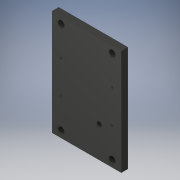
# Autodesk Inventor part: lidarCamMount
Saved by Autodesk Inventor 2017 (Build 210142000, 142)
## iProperties
Created: 2017-03-03
Part Number: lidarCamMount
Material: Polyethylene, High Density
Document SubType Name: Modeling
Designer: Naga
Density: 0.952 g/cm^3
Appearance: Smooth - Black
Author: Naga
Autodesk Inventor part; units mm, degrees
ref_plane "YZ Plane" through (0, 0, 0) normal (1, 0, 0) x (0, 1, 0)
ref_plane "XZ Plane" through (0, 0, 0) normal (0, 1, 0) x (-1, 0, 0)
ref_plane "XY Plane" through (0, 0, 0) normal (0, 0, 1) x (1, 0, 0)
sketch "Sketch1" plane through (0, 0, 0) normal (0, 0, 1) x (1, 0, 0)
  line L0 (24.6062, -15.875) -> (-24.6062, -15.875)
  line L1 (-24.6062, -15.875) -> (-24.6062, 15.875)
  line L2 (-24.6062, 15.875) -> (24.6062, 15.875)
  line L3 (24.6062, 15.875) -> (24.6062, -15.875)
  line L4 (24.6062, -15.875) -> (-24.6062, 15.875) construction
  line L5 (-24.6062, -15.875) -> (24.6062, 15.875) construction
  circle A0 centre (24.6062, 15.875) radius 0.7937
  circle A1 centre (-24.6062, 15.875) radius 0.7937
  circle A2 centre (24.6062, -15.875) radius 0.7937
  circle A3 centre (-24.6062, -15.875) radius 0.7937
  line L6 (-24.6062, -15.875) -> (-24.6062, -22.225)
  line L7 (-24.6062, -15.875) -> (-30.9563, -15.875)
  line L8 (-30.9563, -22.225) -> (32.5437, -22.225)
  line L9 (32.5437, -22.225) -> (32.5437, 31.75)
  line L10 (32.5437, 31.75) -> (-30.9563, 31.75)
  line L11 (-30.9563, 31.75) -> (-30.9563, -22.225)
  line L12 (24.6062, 15.875) -> (-12.2237, 15.875)
  line L13 (-30.9563, 31.75) -> (-30.9563, -22.225)
  line L14 (-24.6062, 15.875) -> (12.2237, 15.875)
  line L15 (12.2237, 15.875) -> (12.2237, -20.955)
  line L16 (12.2237, -20.955) -> (-24.6062, -20.955)
  line L17 (-24.6062, -20.955) -> (-24.6062, 15.875)
  circle A4 centre (12.2237, -20.955) radius 0.7937
  line L18 (-24.6062, 15.875) -> (-24.6062, 44.45)
  line L19 (24.6062, -15.875) -> (24.6062, -44.45)
  circle A5 centre (24.6062, -44.45) radius 3.175
  circle A6 centre (-24.6062, 44.45) radius 3.175
  line L20 (33.3375, -50.8) -> (-33.3375, -50.8)
  line L21 (-33.3375, -50.8) -> (-33.3375, 50.8)
  line L22 (-33.3375, 50.8) -> (33.3375, 50.8)
  line L23 (33.3375, 50.8) -> (33.3375, -50.8)
  line L24 (33.3375, -50.8) -> (-33.3375, 50.8) construction
  line L25 (-33.3375, -50.8) -> (33.3375, 50.8) construction
  point P0 (0, 0)
  dimension "d0" = 49.2125
  dimension "d1" = 31.75
  dimension "d2" = 1.5875
  dimension "d5" = 49.2125
  dimension "d8" = 31.75
  dimension "d11" = 6.35
  dimension "d12" = 6.35
  dimension "d13" = 63.5
  dimension "d14" = 53.975
  dimension "d25" = 36.83
  dimension "d26" = 36.83
  dimension "d27" = 1.5875
  dimension "d28" = 28.575
  dimension "d29" = 28.575
  dimension "d30" = 6.35
  dimension "d31" = 6.35
  dimension "d32" = 66.675
  dimension "d33" = 101.6
  constraints: 52 end point, 8 parallel, 7 centre point, 6 horizontal, 5 perpendicular, 4 coincident, 4 midpoint, 2 point on line, 2 vertical, 6 other
  measures "d0" distance of L1.end L2.end
  measures "d1" distance of L0.end L1.end
  measures "d2" diameter of A0
  measures "d5" distance of L12.start L14.start
  measures "d8" distance of L12.start L19.start
  measures "d11" distance of L6.start L6.end
  measures "d12" distance of L6.start L7.end
  measures "d13" distance of L10.end L9.end
  measures "d14" distance of L9.end L8.end
  measures "d25" distance of L15.end L16.end
  measures "d26" distance of L14.end L15.end
  measures "d27" diameter of A4
  measures "d28" distance of L14.start L18.end
  measures "d29" distance of L19.start L19.end
  measures "d30" diameter of A5
  measures "d31" diameter of A6
  measures "d32" distance of L21.end L22.end
  measures "d33" distance of L20.end L21.end
sketch "Sketch3" plane through (0, 0, 0) normal (0, 0, 1) x (1, 0, 0)
  line L0 (24.6062, -15.875) -> (-24.6062, -15.875)
  line L1 (-24.6062, -15.875) -> (-24.6062, 15.875)
  line L2 (-24.6062, 15.875) -> (24.6062, 15.875)
  line L3 (24.6062, 15.875) -> (24.6062, -15.875)
  line L4 (24.6062, -15.875) -> (-24.6062, 15.875) construction
  line L5 (-24.6062, -15.875) -> (24.6062, 15.875) construction
  circle A0 centre (24.6062, 15.875) radius 0.7937
  circle A1 centre (-24.6062, 15.875) radius 0.7937
  circle A2 centre (24.6062, -15.875) radius 0.7937
  circle A3 centre (-24.6062, -15.875) radius 0.7937
  line L6 (-24.6062, -15.875) -> (-24.6062, -22.225)
  line L7 (-24.6062, -15.875) -> (-30.9563, -15.875)
  line L8 (-30.9563, -22.225) -> (32.5437, -22.225)
  line L9 (32.5437, -22.225) -> (32.5437, 31.75)
  line L10 (32.5437, 31.75) -> (-30.9563, 31.75)
  line L11 (-30.9563, 31.75) -> (-30.9563, -22.225)
  line L12 (24.6062, 15.875) -> (-12.2237, 15.875)
  line L13 (-30.9563, 31.75) -> (-30.9563, -22.225)
  line L14 (-24.6062, 15.875) -> (12.2237, 15.875)
  line L15 (12.2237, 15.875) -> (12.2237, -20.955)
  line L16 (12.2237, -20.955) -> (-24.6062, -20.955)
  line L17 (-24.6062, -20.955) -> (-24.6062, 15.875)
  circle A4 centre (12.2237, -20.955) radius 0.7937
  line L18 (-24.6062, 15.875) -> (-24.6062, 44.45)
  line L19 (24.6062, -15.875) -> (24.6062, -44.45)
  circle A5 centre (24.6062, -44.45) radius 3.175
  circle A6 centre (-24.6062, 44.45) radius 3.175
  line L20 (33.3375, -50.8) -> (-33.3375, -50.8)
  line L21 (-33.3375, -50.8) -> (-33.3375, 50.8)
  line L22 (-33.3375, 50.8) -> (33.3375, 50.8)
  line L23 (33.3375, 50.8) -> (33.3375, -50.8)
  line L24 (33.3375, -50.8) -> (-33.3375, 50.8) construction
  line L25 (-33.3375, -50.8) -> (33.3375, 50.8) construction
  point P0 (0, 0)
  dimension "d34" = 49.2125
  dimension "d35" = 31.75
  dimension "d36" = 1.5875
  dimension "d37" = 49.2125
  dimension "d38" = 31.75
  dimension "d39" = 6.35
  dimension "d40" = 6.35
  dimension "d41" = 63.5
  dimension "d42" = 53.975
  dimension "d43" = 36.83
  dimension "d44" = 36.83
  dimension "d45" = 1.5875
  dimension "d46" = 28.575
  dimension "d47" = 28.575
  dimension "d48" = 6.35
  dimension "d49" = 6.35
  dimension "d50" = 66.675
  dimension "d51" = 101.6
  constraints: 52 end point, 8 parallel, 7 centre point, 6 horizontal, 5 perpendicular, 4 coincident, 4 midpoint, 2 point on line, 2 vertical, 6 other
  measures "d34" distance of L1.end L2.end
  measures "d35" distance of L0.end L1.end
  measures "d36" diameter of A0
  measures "d37" distance of L12.start L14.start
  measures "d38" distance of L12.start L19.start
  measures "d39" distance of L6.start L6.end
  measures "d40" distance of L6.start L7.end
  measures "d41" distance of L10.end L9.end
  measures "d42" distance of L9.end L8.end
  measures "d43" distance of L15.end L16.end
  measures "d44" distance of L14.end L15.end
  measures "d45" diameter of A4
  measures "d46" distance of L14.start L18.end
  measures "d47" distance of L19.start L19.end
  measures "d48" diameter of A5
  measures "d49" diameter of A6
  measures "d50" distance of L21.end L22.end
  measures "d51" distance of L20.end L21.end
extrude "Extrusion2" add sketch "Sketch1" along normal blind 6.35 contours A3 L6 L0 | A3 L1 A1 L2 L15 L0 | L0 L1 A3 | L0 L15 A4 L16 L6 A3 | L7 A3 L1 | L6 A3 L7 | L15 L2 A0 L3 A2 L0 | L0 A2 L19 L8 L6 L16 A4 L15 | A3 L7 L11 L10 L18 A1 L1 | L6 L8 L11 L7 A3 | A2 L3 L0 | L0 L19 A2 | L2 A1 L18 L10 L9 L8 L19 A2 L3 A0 | A4 L16 L15 | L15 L16 A4 | A1 L18 L1 | L1 L2 A1 | L3 A2 L19 | A0 L3 L2 | L2 L3 A0 | L18 A1 L2 | L20 L21 L22 L23
extrude "Extrusion3" cut sketch "Sketch3" along normal blind 6.35 contours A3 L6 L0 | L0 L1 A3 | L7 A3 L1 | L6 A3 L7 | A2 L3 L0 | L0 L19 A2 | A4 L16 L15 | L15 L16 A4 | A1 L18 L1 | L1 L2 A1 | L3 A2 L19 | A0 L3 L2 | L2 L3 A0 | L18 A1 L2
sketch "Sketch7" plane through (0, 0, 0) normal (0, 0, -1) x (-1, 0, 0)
  circle A0 centre (-24.6062, 15.875) radius 0.7937 projected
  circle A1 centre (-12.2237, -20.955) radius 0.7937 projected
  circle A2 centre (24.6062, -15.875) radius 0.7937 projected
  circle A3 centre (24.6062, 15.875) radius 0.7937 projected
  circle A4 centre (-24.6062, -15.875) radius 0.7937 projected
  line L0 (-21.8566, 15.875) -> (-23.2314, 13.4938)
  line L1 (-23.2314, 13.4938) -> (-25.9811, 13.4938)
  line L2 (-25.9811, 13.4938) -> (-27.3559, 15.875)
  line L3 (-27.3559, 15.875) -> (-25.9811, 18.2562)
  line L4 (-25.9811, 18.2562) -> (-23.2314, 18.2563)
  line L5 (-23.2314, 18.2563) -> (-21.8566, 15.875)
  line L6 (-21.8566, -15.875) -> (-23.2314, -18.2562)
  line L7 (-23.2314, -18.2562) -> (-25.9811, -18.2562)
  line L8 (-25.9811, -18.2562) -> (-27.3559, -15.875)
  line L9 (-27.3559, -15.875) -> (-25.9811, -13.4937)
  line L10 (-25.9811, -13.4937) -> (-23.2314, -13.4937)
  line L11 (-23.2314, -13.4937) -> (-21.8566, -15.875)
  line L12 (26.9875, -15.875) -> (25.7969, -17.9372)
  line L13 (25.7969, -17.9372) -> (23.4156, -17.9372)
  line L14 (23.4156, -17.9372) -> (22.225, -15.875)
  line L15 (22.225, -15.875) -> (23.4156, -13.8128)
  line L16 (23.4156, -13.8128) -> (25.7969, -13.8128)
  line L17 (25.7969, -13.8128) -> (26.9875, -15.875)
  point P0 (0, 0)
  dimension "d118" = 4.7625
  dimension "d119" = 4.7625
  dimension "d120" = 4.7625
  constraints: 36 end point, 3 coincident, 39 other
  measures "d118" distance between parallel lines of L1 L4
  measures "d119" distance of L12.start L14.end
  measures "d120" distance from line of L9 L6.start
extrude "Extrusion4" cut sketch "Sketch7" against normal blind 1.5875 contours L0 L1 L2 L3 L4 L5 | L6 L7 L8 L9 L10 L11 | L12 L13 L14 L15 L16 L17
sketch "Sketch8" plane through (0, 0, 6.35) normal (0, 0, 1) x (1, 0, 0)
  circle A0 centre (12.2237, -20.955) radius 0.7937 projected
  circle A1 centre (12.2237, -20.955) radius 2.3813
  point P0 (0, 0)
  dimension "d123" = 4.7625
  constraints: 1 centre point, 1 coincident
  measures "d123" diameter of A1
extrude "Extrusion5" cut sketch "Sketch8" against normal blind 3.175
sketch "Sketch9" plane through (0, 0, 6.35) normal (0, 0, 1) x (1, 0, 0)
  circle A0 centre (24.6062, -44.45) radius 3.175 projected
  circle A1 centre (-24.6062, 44.45) radius 3.175 projected
  line L0 (-24.6062, 44.45) -> (24.6062, 44.45)
  line L1 (24.6062, 44.45) -> (24.6062, -44.45)
  line L2 (24.6062, -44.45) -> (-24.6062, -44.45)
  line L3 (-24.6062, -44.45) -> (-24.6062, 44.45)
  circle A2 centre (-24.6062, -44.45) radius 3.175
  circle A3 centre (24.6062, 44.45) radius 3.175
  point P0 (0, 0)
  dimension "d126" = 6.35
  dimension "d127" = 6.35
  constraints: 8 end point, 2 centre point, 2 coincident, 2 parallel, 1 horizontal, 1 perpendicular
  measures "d126" diameter of A2
  measures "d127" diameter of A3
extrude "Extrusion6" cut sketch "Sketch9" against normal blind 6.35 contours A3 L0 L1 | L1 L0 A3 | A2 L3 L2 | L2 L3 A2
body "Solid2"
